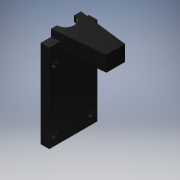
# Autodesk Inventor part: LearnbotSupportCameraC
Saved by Autodesk Inventor 2017 (Build 210142000, 142)
## iProperties
Part Number: LearnbotSupportCameraC
Material: Genérico
Document SubType Name: Modeling
Designer: Roberto
Density: 1 g/cm^3
Appearance: Valor por defecto
Author: Roberto
Autodesk Inventor part; units mm, degrees
ref_plane "YZ Plane" through (0, 0, 0) normal (1, 0, 0) x (0, 1, 0)
ref_plane "XZ Plane" through (0, 0, 0) normal (0, 1, 0) x (-1, 0, 0)
ref_plane "XY Plane" through (0, 0, 0) normal (0, 0, 1) x (1, 0, 0)
sketch "Boceto1" plane through (0, 0, 0) normal (0, 0, 1) x (1, 0, 0)
  arc A0 (1.4408, -0.1992) -> (1.4375, 0.1994) centre (1.4226, 0) ccw
  line L0 (0.2295, 0.2896) -> (1.4375, 0.1994)
  line L1 (0.1967, -0.3128) -> (1.4408, -0.1992)
  arc A1 (0, -0.3) -> (0, 0.3) centre (0, 0) ccw
  line L2 (0, 0) -> (0, 0.55)
  line L3 (1.7726, 0.3309) -> (0, 0.55)
  line L4 (1.7726, -0.3258) -> (0, -0.5087)
  line L5 (1.6226, 0.0017) -> (1.7726, 0.0017)
  line L6 (1.7726, 0.0017) -> (1.7726, 0.3309)
  line L7 (1.7726, 0.3309) -> (1.7726, -0.3258)
  line L8 (0, 0.55) -> (0, -0.5087)
  arc A2 (0.2295, 0.2896) -> (0, 0.3695) centre (0, 0) ccw
  arc A3 (0, -0.3695) -> (0.1967, -0.3128) centre (0, 0) ccw
  line L9 (0, 0.3) -> (0, -0.3)
  constraints: 20 end point, 9 point on circle, 4 centre point, 4 point on line, 3 vertical, 1 horizontal, 1 perpendicular
extrude "Extrusión1" add sketch "Boceto1" along normal blind 0.2 contours L1 A3 L8 A1 L2 A2 L0 A0 | A0 L5 L7 L4 L8 A3 L1 | A0 L0 A2 L2 L3 L6 L5
sketch "Boceto2" plane through (0, 0, 0) normal (0, 0, -1) x (-1, 0, 0)
  line L0 (0, 0) -> (0, 0.55)
  line L1 (0, 0.55) -> (0, -0.5087)
  line L2 (0, 0.3) -> (0, -0.3)
  line L3 (0, 0) -> (0, 0.55)
  line L4 (0, 0.55) -> (0, -0.5087)
  line L5 (0, 0.3) -> (0, -0.3)
  arc A0 (0, 0.3) -> (0, -0.3) centre (0, 0) ccw
  arc A1 (-0.1967, -0.3128) -> (0, -0.3695) centre (0, 0) ccw
  line L6 (-0.2295, 0.2896) -> (-1.4375, 0.1994)
  line L7 (-0.1967, -0.3128) -> (-1.4408, -0.1992)
  arc A2 (-1.4375, 0.1994) -> (-1.4408, -0.1992) centre (-1.4226, 0) ccw
  line L8 (-1.7726, -0.3258) -> (0, -0.5087)
  line L9 (-1.7726, 0.3309) -> (-1.7726, -0.3258)
  line L10 (-1.7726, 0.0017) -> (-1.7726, 0.3309)
  line L11 (-1.6226, 0.0017) -> (-1.7726, 0.0017)
  line L12 (-1.7726, 0.3309) -> (0, 0.55)
  arc A3 (0, 0.3695) -> (-0.2295, 0.2896) centre (0, 0) ccw
  arc A4 (0, 0.3) -> (0, -0.3) centre (0, 0) ccw
  arc A5 (-0.1967, -0.3128) -> (0, -0.3695) centre (0, 0) ccw
  line L13 (-0.2295, 0.2896) -> (-1.4375, 0.1994)
  line L14 (-0.1967, -0.3128) -> (-1.4408, -0.1992)
  arc A6 (-1.4375, 0.1994) -> (-1.4408, -0.1992) centre (-1.4226, 0) ccw
  line L15 (-1.7726, -0.3258) -> (0, -0.5087)
  line L16 (-1.7726, 0.3309) -> (-1.7726, -0.3258)
  line L17 (-1.7726, 0.0017) -> (-1.7726, 0.3309)
  line L18 (-1.6226, 0.0017) -> (-1.7726, 0.0017)
  line L19 (-1.7726, 0.3309) -> (0, 0.55)
  arc A7 (0, 0.3695) -> (-0.2295, 0.2896) centre (0, 0) ccw
  constraints: 40 end point, 16 point on circle, 8 centre point, 8 point on line, 6 vertical
extrude "Extrusión2" add sketch "Boceto2" along normal blind 0.15 contours A3 L6 A2 L11 L9 L12 L0 | L1 L8 L9 L11 A2 L7 A1
sketch "Boceto3" plane through (0, 0, -0.15) normal (0, 0, -1) x (-1, 0, 0)
  arc A0 (0, 0.3695) -> (-0.2295, 0.2896) centre (0, 0) ccw projected
  line L0 (-0.2295, 0.2896) -> (-1.4375, 0.1994) projected
  arc A1 (-1.4375, 0.1994) -> (-1.4408, -0.1992) centre (-1.4226, 0) ccw projected
  line L1 (-1.4408, -0.1992) -> (-0.1967, -0.3128) projected
  arc A2 (-0.1967, -0.3128) -> (0, -0.3695) centre (0, 0) ccw projected
  line L2 (0, -0.3) -> (0, -0.3695) projected
  line L3 (0, -0.5087) -> (0, -0.3695) projected
  arc A3 (-0.1967, -0.3128) -> (0, -0.3695) centre (0, 0) ccw projected
  line L4 (-0.1967, -0.3128) -> (-1.4408, -0.1992) projected
  arc A4 (-1.4375, 0.1994) -> (-1.4408, -0.1992) centre (-1.4226, 0) ccw projected
  line L5 (-1.4375, 0.1994) -> (-0.2295, 0.2896) projected
  arc A5 (0, 0.3695) -> (-0.2295, 0.2896) centre (0, 0) ccw projected
  line L6 (0, 0.3695) -> (0, 0.55) projected
  line L7 (0, 0.55) -> (-1.7726, 0.3309) projected
  line L8 (-1.7726, 0.3309) -> (-1.7726, -0.3258) projected
  line L9 (-1.7726, -0.3258) -> (0, -0.5087) projected
  arc A6 (0, 0.3) -> (0, -0.3) centre (0, 0) ccw projected
  line L10 (0, 0.3695) -> (0, 0.3) projected
extrude "Extrusión3" add sketch "Boceto3" along normal blind 0.2
sketch "Boceto4" plane through (0, 0, -0.35) normal (0, 0, -1) x (-1, 0, 0)
  line L0 (0, -0.5087) -> (0, 0.55) projected
  line L1 (-1.7726, 0.3309) -> (0, 0.55) projected
  line L2 (0, 0.55) -> (0, 0.83)
  line L3 (0, 0.83) -> (-0.3, 0.83)
  line L4 (-0.3, 0.83) -> (-0.3, -0.87)
  line L5 (-0.3, -0.87) -> (0, -0.87)
  line L6 (0, -0.87) -> (0, 0.83)
  point P0 (0, 0)
  dimension "d8" = 0.28
  dimension "d9" = 0.3
  dimension "d10" = 1.7
  constraints: 10 end point, 3 perpendicular, 1 horizontal, 1 vertical
  measures "d8" distance of L0.end L2.end
  measures "d9" distance of L2.end L3.end
  measures "d10" distance of L3.end L4.end
extrude "Extrusión4" add sketch "Boceto4" along normal blind 2.8 and the other way blind 0.1
sketch "Boceto5" plane through (0.3, -0.4778, -0.35) normal (1, 0, 0) x (0, 0, -1)
  line L0 (0, -0.3922) -> (2.3, -0.3922)
  line L1 (0, -0.3922) -> (0, 1.1078)
  line L2 (0, 1.3078) -> (0, -0.3922)
  line L3 (0, -0.3922) -> (0, -0.1922)
  line L4 (0, 1.3078) -> (2.3, 1.3078)
  line L5 (-0.1, 0.9907) -> (-0.1, 1.3078) projected
  line L6 (0, 0.9907) -> (0, 0.8087) projected
  line L7 (0, 0.9907) -> (0, 1.3078)
  circle A0 centre (0.3, 1.1078) radius 0.1
  circle A1 centre (0.3, -0.1922) radius 0.1
  circle A2 centre (2.46, 1.1078) radius 0.1
  circle A3 centre (2.46, -0.1922) radius 0.1
  line L8 (2.46, 1.1078) -> (2.46, 1.1492)
  point P0 (-0.35, 0.4778)
  dimension "d15" = 0.2
  dimension "d27" = 0.2
  constraints: 14 end point, 4 centre point, 2 point on line, 2 vertical
  measures "d15" distance of L2.end L3.end
  measures "d27" diameter of A1
extrude "Extrusión5" cut sketch "Boceto5" against normal blind 2.3
sketch "Boceto6" plane through (0, 0, -0.25) normal (0, 0, 1) x (1, 0, 0)
  line L0 (0, -0.5087) -> (0.3, -0.4778) projected
  line L1 (0, -0.5087) -> (0, -0.87) projected
  line L2 (0, -0.87) -> (0.3, -0.87) projected
  line L3 (0.3, -0.87) -> (0.3, -0.4778) projected
  line L4 (0.3, 0.5129) -> (0, 0.55) projected
  line L5 (0.3, 0.5129) -> (0.3, 0.83) projected
  line L6 (0.3, 0.83) -> (0, 0.83) projected
  line L7 (0, 0.83) -> (0, 0.55) projected
  point P0 (0, 0)
extrude "Extrusión6" add sketch "Boceto6" along normal blind 0.2
